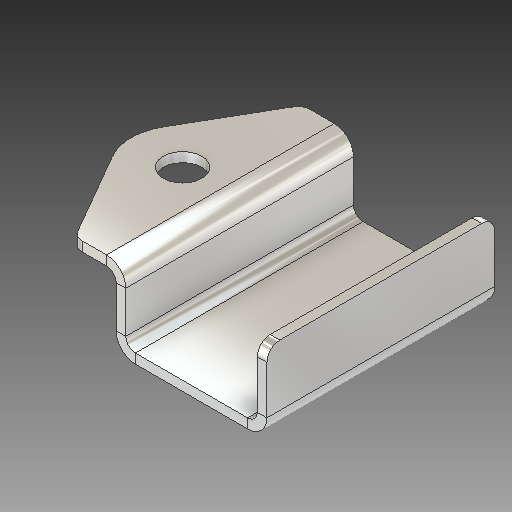
# Autodesk Inventor part: 318-02
Saved by Autodesk Inventor 2019 (Build 230136000, 136)
## iProperties
Company: Autodesk Inc.
Created: 2017-07-21
Part Number: 318-02
Material: Aluminum 6061
Document SubType Name: Sheet Metal
Designer: Autodesk Inc.
Mass: 61.1477 g
Surface Area: 162.401 cm^2
Volume: 22.6473 cm^3
Density: 2.7 g/cm^3
Sheet Metal Rule: Default_mm
Appearance: Chrome - Polished
Description: RAIL SLIDE
Author: Inventor
Autodesk Inventor part; units mm, degrees
ref_plane "YZ Plane" through (0, 0, 0) normal (1, 0, 0) x (0, 1, 0)
ref_plane "XZ Plane" through (0, 0, 0) normal (0, 1, 0) x (-1, 0, 0)
ref_plane "XY Plane" through (0, 0, 0) normal (0, 0, 1) x (1, 0, 0)
sketch "Sketch1" plane through (0, 0, 0) normal (0, 1, 0) x (-1, 0, 0)
  line L0 (-20.5, 35.5) -> (20.5, 35.5)
  line L1 (20.5, 35.5) -> (20.5, -35.5)
  line L2 (20.5, -35.5) -> (-20.5, -35.5)
  line L3 (-20.5, -35.5) -> (-20.5, 35.5)
  line L4 (-20.5, 35.5) -> (20.5, -35.5) construction
  line L5 (20.5, 35.5) -> (-20.5, -35.5) construction
  point P0 (0, 0)
  point P1 (0, 0)
  point P2 (0, 0)
  dimension "d0" = 71
  dimension "d1" = 41
  measures "d0" distance of L0.end L1.end
  measures "d1" distance of L1.end L2.end
extrude "Plate1" add sketch "Sketch1" along normal blind 3
sketch "Sketch2" plane through (20.5, 3, -35.5) normal (1, 0, 0) x (0, 1, 0)
  line L0 (0, 71) -> (0, 0)
  line L1 (0, 0) -> (22, 0)
  line L2 (22, 0) -> (22, 71)
  line L3 (22, 71) -> (0, 71)
  constraints: 6 end point, 1 horizontal, 1 perpendicular, 1 vertical
edge flange "Flange1" height 22 angle 90 thickness 3 bend radius 3 thickness toward (1, 0, 0) relief tear relief width 3 relief depth 1.5 corner gap 3 corner form 0 edges at (20.5, 3, 0) (-20.5, 3, 0) wall of the first edge with corners at (20.5, 3, 35.5) (20.5, 3, -35.5) (20.5, 25, -35.5) (20.5, 25, 35.5)
bend "Bend1"
corner "Corner1"
sketch "Sketch3" plane through (-20.5, 22, -35.5) normal (0, 1, 0) x (-1, 0, 0)
  line L0 (0, 71) -> (0, 0)
  line L1 (0, 0) -> (33.8, 0)
  line L2 (33.8, 0) -> (33.8, 71)
  line L3 (33.8, 71) -> (0, 71)
  constraints: 6 end point, 1 horizontal, 1 perpendicular, 1 vertical
edge flange "Flange2" height 33.8 angle 90 thickness 3 bend radius 3 thickness toward (0, 1, 0) relief tear relief width 3 relief depth 1.5 edges at (-23.5, 25, 0) wall of the first edge with corners at (-20.5, 22, 35.5) (-20.5, 22, -35.5) (-54.3, 22, -35.5) (-54.3, 22, 35.5)
bend "Bend2"
corner "Corner2"
sketch "Sketch4" plane through (-54.3, 25, 35.5) normal (0, 1, 0) x (1, 0, 0)
  line L0 (0, 0) -> (28.3, 0)
  line L1 (28.3, 71) -> (0, 71)
  line L2 (0, 0) -> (0, 71)
  line L3 (54.3, 35.5) -> (0, 35.5) construction
  line L4 (2.1436, 27.5) -> (18.0207, 0)
  line L5 (2.1436, 43.5) -> (18.0207, 71)
  arc A0 (2.1436, 43.5) -> (2.1436, 27.5) centre (16, 35.5) ccw
  line L6 (74.8, 71) -> (77.8, 71) projected
  line L7 (74.8, 0) -> (77.8, 0) projected
  point P0 (54.3, 35.5)
  dimension "d23" = 30
  dimension "d24" = 30
  dimension "d25" = 16
  dimension "d26" = 38.3
  constraints: 12 end point, 3 point on circle, 3 point on line, 2 collinear, 2 tangent, 1 centre point, 1 coincident, 1 horizontal, 1 midpoint, 1 vertical
  measures "d23" angle of L2 L4
  measures "d24" angle of L2 L5
  measures "d25" radius of A0
  measures "d26" distance of point (54.3, 35.5) A0.centre
extrude "Cut1" cut sketch "Sketch4" against normal blind 3
fillet "Fillet1" radius 4 4 edges at (-36.2793, 23.5, 35.5) (-36.2793, 23.5, -35.5) (22, 25, -35.5) (22, 25, 35.5)
sketch "Sketch5" plane through (-26.5, 25, 35.5) normal (0, 1, 0) x (1, 0, 0)
  arc A0 (-25.6564, 43.5) -> (-25.6564, 27.5) centre (-11.8, 35.5) ccw projected
  circle A1 centre (-11.8, 35.5) radius 6
  point P0 (26.5, 35.5)
  dimension "d30" = 12
  constraints: 1 centre point, 1 coincident
  measures "d30" diameter of A1
extrude "Extrusion1" cut sketch "Sketch5" against normal through all
equation "\"d24\" = d23"
equation "\"d27\" = Thickness"
equation "\"d2\" = Thickness"
equation "\"d3\" = BendReliefWidth"
equation "\"d4\" = BendReliefDepth"
equation "\"d5\" = MinimumRemnant"
equation "\"d6\" = TransitionRadius"
equation "\"d9\" = BendRadius"
equation "\"d10\" = CornerReliefSize"
equation "\"d11\" = GapSize"
equation "\"d12\" = JacobiRadiusSize"
equation "\"d13\" = BendReliefWidth"
equation "\"d14\" = BendReliefDepth"
equation "\"d15\" = MinimumRemnant"
equation "\"d16\" = TransitionRadius"
equation "\"d19\" = BendRadius"
equation "\"d20\" = CornerReliefSize"
equation "\"d21\" = GapSize"
equation "\"d22\" = JacobiRadiusSize"
equation "\"BendRadius\" = Thickness"
equation "\"BendReliefWidth\" = Thickness"
equation "\"BendReliefDepth\" = 0.5 * Thickness"
equation "\"CornerReliefSize\" = 4 * Thickness"
equation "\"MinimumRemnant\" = 2 * Thickness"
equation "\"TransitionRadius\" = BendRadius"
equation "\"JacobiRadiusSize\" = BendRadius"
equation "\"GapSize\" = Thickness"
equation "\"Thickness\" = 3"
body "Solid1"
